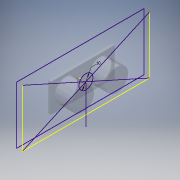
# Autodesk Inventor part: Ultrasound
Saved by Autodesk Inventor 2017 (Build 210142000, 142)
## iProperties
Created: 2020-08-23
Part Number: Ultrasound
Material: PET Plastic
Document SubType Name: Modeling
Designer: agustin
Density: 1.541 g/cm^3
Appearance: Polycarbonate - Clear
Author: agustin
Autodesk Inventor part; units mm, degrees
ref_plane "YZ Plane" through (0, 0, 0) normal (1, 0, 0) x (0, 1, 0)
ref_plane "XZ Plane" through (0, 0, 0) normal (0, 1, 0) x (-1, 0, 0)
ref_plane "XY Plane" through (0, 0, 0) normal (0, 0, 1) x (1, 0, 0)
sketch "Sketch1" plane through (0, 0, 0) normal (1, 0, 0) x (0, 1, 0)
  line L0 (-20.4, 45.3) -> (20.4, 45.3)
  line L1 (20.4, 45.3) -> (20.4, -45.3)
  line L2 (20.4, -45.3) -> (-20.4, -45.3)
  line L3 (-20.4, -45.3) -> (-20.4, 45.3)
  line L4 (-20.4, 45.3) -> (20.4, -45.3) construction
  line L5 (20.4, 45.3) -> (-20.4, -45.3) construction
  point P0 (0, 0)
  dimension "d0" = 40.8
  dimension "d1" = 90.6
  constraints: 12 end point, 2 midpoint, 2 parallel, 1 horizontal, 1 perpendicular
  measures "d0" distance of L1.end L2.end
  measures "d1" distance of L0.end L1.end
extrude "Extrusion1" add sketch "Sketch1" along normal blind 4
sketch "Sketch2" plane through (4, 0, 0) normal (1, 0, 0) x (0, 0, -1)
  circle A0 centre (-24.3, 0) radius 16
  line L0 (-45.3, 20.4) -> (-45.3, -20.4) projected
  line L1 (-45.3, 0) -> (-40.3, 0)
  line L2 (-45.3, 0) -> (-41.0258, 0)
  line L3 (45.3, 20.4) -> (-45.3, 20.4) projected
  line L4 (-45.3, -20.4) -> (45.3, -20.4) projected
  circle A1 centre (24.3, 0) radius 16
  dimension "d4" = 32
  constraints: 4 end point, 2 centre point, 1 horizontal, 1 midpoint, 1 point on line
  measures "d4" diameter of A0
extrude "Extrusion2" add sketch "Sketch2" along normal blind 24
sketch "Sketch3" plane through (4, 0, 0) normal (1, 0, 0) x (0, 0, -1)
  line L0 (-45.3, 20.4) -> (-45.3, -20.4) projected
  line L1 (-45.3, -20.4) -> (45.3, -20.4) projected
  line L2 (-45.3, 20.4) -> (45.3, -20.4)
  line L3 (45.3, -20.4) -> (45.3, 20.4) projected
  line L4 (-45.3, -20.4) -> (45.3, 20.4)
  circle A0 centre (0, 0) radius 5
  line L5 (0, 0) -> (0, -27.8597)
  dimension "d9" = 10
  constraints: 6 end point, 1 centre point, 1 coincident, 1 vertical
  measures "d9" diameter of A0
sketch "Sketch4" plane through (0, 0, 0) normal (-1, 0, 0) x (0, 0, 1)
  line L0 (-45.3, -20.4) -> (-45.3, 20.4) projected
  line L1 (45.3, 20.4) -> (45.3, -20.4) projected
  line L2 (-45.3, 20.4) -> (45.3, 20.4)
  line L3 (45.3, 20.4) -> (45.3, -20.4)
  line L4 (45.3, -20.4) -> (-45.3, -20.4)
  line L5 (-45.3, -20.4) -> (-45.3, 20.4)
  point P0 (0, 0)
  constraints: 8 end point, 2 parallel, 1 horizontal, 1 perpendicular
scale "Scale1" factors (0.5, 0.5, 0.5) then translate (0, 0, 0) bodies 1
body "Solid1"
